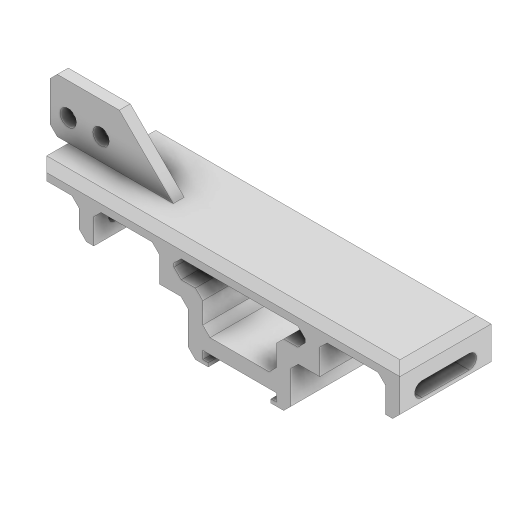
# Autodesk Inventor part: adapter_ver.1
Saved by Autodesk Inventor 2024 (Build 280153000, 153)
## iProperties
Created: 2023-11-09
Part Number: adapter_ver.1
Material: 一般
Document SubType Name: Modeling
Designer: moonshot
Density: 1 g/cm^3
Appearance: 既定
Author: moonshot
Autodesk Inventor part; units mm, degrees
ref_plane "YZ Plane" through (0, 0, 0) normal (1, 0, 0) x (0, 1, 0)
sketch "スケッチ1" plane through (0, 0, 0) normal (0, 0, 1) x (1, 0, 0)
  line L0 (94.5, 17.4061) -> (94.5, 4.4383)
  line L1 (64.6, 4.4061) -> (64.6, -8.5939)
  line L2 (36.4, -8.5939) -> (36.4, 4.4061)
  line L3 (0, -17.7867) -> (0, 46.5626) projected
  line L4 (40.4, -5.3939) -> (60.6, -5.3939)
  line L5 (64.6, -8.5939) -> (59.1, -8.5939)
  line L6 (41.9, -8.5939) -> (36.4, -8.5939)
  line L7 (72.5, 4.4061) -> (72.5, 13.4061)
  line L8 (72.5, 13.4061) -> (90.5, 13.4061)
  line L9 (90.5, 13.4061) -> (90.5, 4.4383)
  line L10 (50.5, -8.5617) -> (50.5, 17.1682) construction
  line L11 (28.5, 4.4061) -> (28.5, 13.4061)
  line L12 (28.5, 13.4061) -> (10.5, 13.4061)
  line L13 (10.5, 13.4061) -> (10.5, 4.4383)
  line L14 (0, 17.4061) -> (0, 13.4061)
  line L15 (0, 17.4061) -> (94.5, 17.4061)
  line L16 (94.5, 4.4383) -> (90.5, 4.4383)
  line L17 (72.5, 4.4061) -> (64.6, 4.4061)
  line L18 (6.5, 4.4383) -> (10.5, 4.4383)
  line L19 (28.5, 4.4061) -> (36.4, 4.4061)
  line L20 (6.5, 4.4383) -> (6.5, 13.4061)
  line L21 (6.5, 13.4061) -> (0, 13.4061)
  line L22 (72.5, 4.4061) -> (82.5, 4.4061) construction
  line L23 (82.5, 4.4061) -> (82.5, 13.4061) construction
  line L24 (77.5, 4.4061) -> (77.5, 37.3698) construction
  line L25 (28.5, 4.4061) -> (18.5, 4.4061) construction
  line L26 (18.5, 4.4061) -> (18.5, 13.4061) construction
  line L27 (23.5, 4.4061) -> (23.5, 33.4166) construction
  line L28 (41.9, -8.5939) -> (41.9, -7.5939)
  line L29 (41.9, -7.5939) -> (40.4, -7.5939)
  line L30 (40.4, -7.5939) -> (40.4, -5.3939)
  line L31 (59.1, -8.5939) -> (59.1, -7.5939)
  line L32 (59.1, -7.5939) -> (60.6, -7.5939)
  line L33 (60.6, -7.5939) -> (60.6, -5.3939)
  line L34 (32.5, 13.4061) -> (32.5, 8.4061)
  line L35 (40.4, 8.4061) -> (40.4, -1.3939)
  line L36 (40.4, -1.3939) -> (60.6, -1.3939)
  line L37 (60.6, -1.3939) -> (60.6, 8.4061)
  line L38 (60.6, 8.4061) -> (68.5, 8.4061)
  line L39 (68.5, 8.4061) -> (68.5, 13.4061)
  line L40 (68.5, 13.4061) -> (32.5, 13.4061)
  line L41 (32.5, 8.4061) -> (40.4, 8.4061)
  point P0 (0, 0)
  dimension "d10" = 20.2
  dimension "d14" = 18
  dimension "d18" = 13
  dimension "d23" = 4
  dimension "d40" = 4
  dimension "d41" = 9
  dimension "d42" = 10
  dimension "d43" = 10
  dimension "d44" = 50.5
  dimension "d74" = 4
  dimension "d78" = 1
  dimension "d79" = 2.2
  dimension "d80" = 1.5
  dimension "d81" = 1.5
  dimension "d82" = 1
  dimension "d83" = 23.5
  dimension "d84" = 4
  dimension "d86" = 4
  dimension "d87" = 4
  dimension "d88" = 4
  dimension "d89" = 4
  dimension "d90" = 4
  dimension "d91" = 4
  dimension "d92" = 4
  constraints: 82 end point, 23 perpendicular, 6 horizontal, 5 vertical, 4 symmetric about line, 3 point on line, 2 collinear, 2 midpoint, 2 other
  measures "d10" distance of L4.start L4.end
  measures "d14" distance of L7.end L8.end
  measures "d18" distance of L2.end L2.start
  measures "d23" distance between parallel lines of L0 L9
  measures "d40" distance of L18.start L13.end
  measures "d41" distance of L7.start L7.end
  measures "d42" distance of L7.start L22.end
  measures "d43" distance of L11.start L25.end
  measures "d44" distance between parallel lines of L10 L3
  measures "d74" distance between parallel lines of L21 L15
  measures "d78" distance of L6.start L28.end
  measures "d79" distance between parallel lines of L4 L29
  measures "d80" distance of L28.end L29.end
  measures "d81" distance of L31.end L32.end
  measures "d82" distance of L5.end L31.end
  measures "d83" distance between parallel lines of L27 L3
  measures "d84" distance between parallel lines of L30 L2
  measures "d86" distance between parallel lines of L11 L34
  measures "d87" distance between parallel lines of L2 L35
  measures "d88" distance between parallel lines of L4 L36
  measures "d89" distance between parallel lines of L1 L37
  measures "d90" distance between parallel lines of L7 L39
  measures "d91" distance between parallel lines of L17 L38
  measures "d92" distance between parallel lines of L19 L41
extrude "押し出し1" add sketch "スケッチ1" along normal mid plane 25
chamfer "面取り1" distance 2 angle 45 2 edges at (72.5, 13.4061, 0) (28.5, 13.4061, 0)
sketch "スケッチ4" plane through (94.5, 4.4383, 12.5) normal (1, 0, 0) x (0, 0, -1)
  line L0 (6, 3) -> (19, 3)
  arc A0 (19, 3) -> (19, 7) centre (19, 5) ccw
  line L1 (19, 7) -> (6, 7)
  arc A1 (6, 7) -> (6, 3) centre (6, 5) ccw
  line L2 (25, 12.9678) -> (25, 0) projected
  line L3 (0, 0) -> (0, 12.9678) projected
  line L4 (25, 0) -> (0, 0) projected
  point P0 (12.5, -4.4383)
  dimension "d45" = 4
  dimension "d46" = 6
  dimension "d47" = 6
  dimension "d48" = 3
  constraints: 4 end point, 4 point on circle, 4 tangent, 2 centre point, 2 horizontal
  measures "d45" distance between parallel lines of L0 L1
  measures "d46" distance from line of L2 A0.centre
  measures "d47" distance from line of L3 A1.centre
  measures "d48" distance between parallel lines of L4 L0
extrude "押し出し3" cut sketch "スケッチ4" against normal up to surface (4 mm away)
sketch "スケッチ5" plane through (6.5, 4.4383, 12.5) normal (-1, 0, 0) x (0, 0, 1)
  line L0 (-19, 3) -> (-6, 3) projected
  line L1 (-19, 3) -> (-6, 3)
  arc A0 (-6, 3) -> (-6, 7) centre (-6, 5) ccw
  line L2 (-6, 7) -> (-19, 7) projected
  line L3 (-6, 7) -> (-19, 7)
  arc A1 (-19, 7) -> (-19, 3) centre (-19, 5) ccw
  point P0 (-12.5, -4.4383)
  constraints: 4 end point, 4 point on circle, 4 tangent, 2 centre point, 2 equal length
extrude "押し出し4" cut sketch "スケッチ5" against normal up to surface (4 mm away)
chamfer "面取り4" distance 2 angle 45 20 edges at (90.5, 13.4061, 0) (10.5, 13.4061, 0) (6.5, 13.4061, 0) (64.6, 4.4061, 0) (36.4, 4.4061, 0) (40.4, 8.4061, 0) (32.5, 8.4061, 0) (32.5, 13.4061, 0) (68.5, 13.4061, 0) (68.5, 8.4061, 0) (60.6, 8.4061, 0) (60.6, -1.3939, 0) (40.4, -1.3939, 0) (36.4, -8.5939, 0) (64.6, -8.5939, 0) (94.5, 4.4383, 0) (94.5, 17.4061, 0) (47.25, 17.4061, 12.5) (47.25, 17.4061, -12.5) (6.5, 4.4383, 0)
ref_plane "作業平面1" through (0, 0, 1.5) normal (0, 0, 1) x (1, 0, 0)
sketch "スケッチ6" plane through (0, 0, 1.5) normal (0, 0, 1) x (1, 0, 0)
  line L0 (94.5, 17.4061) -> (0, 17.4061) projected
  line L1 (9.5, 17.4061) -> (-9.5, 17.4061)
  line L2 (-9.5, 17.4061) -> (-9.5, 32.2061)
  line L3 (-9.5, 32.2061) -> (9.5, 32.2061)
  line L4 (9.5, 32.2061) -> (9.5, 17.4061)
  line L5 (0, -5.8812) -> (0, 35.2873) projected
  circle A0 centre (4.5, 23.4061) radius 2.25
  circle A1 centre (-4.5, 23.4061) radius 2.25
  point P0 (0, 0)
  dimension "d57" = 19
  dimension "d58" = 14.8
  dimension "d59" = 4.5
  dimension "d60" = 4.5
  dimension "d61" = 6
  constraints: 8 end point, 3 perpendicular, 2 centre point, 1 collinear, 1 point on line, 1 symmetric about line, 2 other
  measures "d57" distance of L2.end L3.end
  measures "d58" distance of L1.end L2.end
  measures "d59" diameter of A0
  measures "d60" distance from line of L5 A0.centre
  measures "d61" distance from line of L0 A0.centre
extrude "押し出し5" add sketch "スケッチ6" along normal blind 3
ref_plane "作業平面2" through (0, 0, 0.1) normal (0, 0, 1) x (1, 0, 0)
sketch "スケッチ7" plane through (0, 0, 0.1) normal (0, 0, 1) x (1, 0, 0)
  line L0 (-9.5, 17.4061) -> (0, 17.4061) projected
  line L1 (9.5, 17.4061) -> (0, 17.4061) projected
  line L2 (9.5, 17.4061) -> (9.5, 32.2061) projected
  line L3 (9.5, 32.2061) -> (-9.5, 32.2061) projected
  line L4 (-9.5, 32.2061) -> (-9.5, 17.4061) projected
  circle A0 centre (4.5, 23.4061) radius 2.25 projected
  circle A1 centre (-4.5, 23.4061) radius 2.25 projected
  line L5 (0, 13.4061) -> (4.5, 13.4061) projected
  line L6 (0, 17.4061) -> (0, 13.4061) projected
  line L7 (0, 13.4061) -> (0, 17.4061)
  line L8 (0, 17.4061) -> (-9.5, 17.4061)
  line L9 (-9.5, 17.4061) -> (0, 17.4061) projected
  line L10 (-4.4, 13.4061) -> (0, 13.4061)
  line L11 (-4.4, 13.4061) -> (-4.4, 17.4061)
  point P0 (0, 0)
  dimension "d70" = 4.4
  constraints: 8 end point, 2 collinear, 1 perpendicular, 1 point on line
  measures "d70" distance of L10.start L5.start
extrude "押し出し6" add sketch "スケッチ7" along normal up to surface (12.4 mm away) contours L0 L6 L10 L11
chamfer "面取り5" distance 14.8 angle 45 1 edges at (9.5, 17.4061, 3)
sketch "スケッチ8" plane through (0, 0, -12.5) normal (0, 0, -1) x (-1, 0, 0)
  line L0 (-4.5, 13.4061) -> (4.4, 13.4061) projected
  line L1 (-0.05, 13.4061) -> (-4.5, 13.4061)
  line L2 (-4.5, 13.4061) -> (0, 13.4061) projected
  line L3 (0, 13.4061) -> (0, 15.4061) projected
  line L4 (-94.5, 15.4061) -> (-94.5, 6.4383) projected
  line L5 (-92.5, 4.4383) -> (-90.5, 4.4383) projected
  line L6 (-90.5, 4.4383) -> (-90.5, 11.4061) projected
  line L7 (-88.5, 13.4061) -> (-90.5, 11.4061) projected
  line L8 (-88.5, 13.4061) -> (-74.5, 13.4061) projected
  line L9 (-72.5, 11.4061) -> (-72.5, 4.4061) projected
  line L10 (-72.5, 4.4061) -> (-66.6, 4.4061) projected
  line L11 (-64.6, 2.4061) -> (-64.6, -6.5939) projected
  line L12 (-62.6, -8.5939) -> (-59.1, -8.5939) projected
  line L13 (-60.6, -5.3939) -> (-40.4, -5.3939) projected
  line L14 (-41.9, -8.5939) -> (-38.4, -8.5939) projected
  line L15 (-36.4, -6.5939) -> (-36.4, 2.4061) projected
  line L16 (-34.4, 4.4061) -> (-28.5, 4.4061) projected
  line L17 (-28.5, 4.4061) -> (-28.5, 11.4061) projected
  line L18 (-26.5, 13.4061) -> (-12.5, 13.4061) projected
  line L19 (-10.5, 11.4061) -> (-12.5, 13.4061) projected
  line L20 (-10.5, 11.4061) -> (-10.5, 4.4383) projected
  line L21 (-10.5, 4.4383) -> (-8.5, 4.4383) projected
  line L22 (-6.5, 6.4383) -> (-6.5, 11.4061) projected
  line L23 (-4.5, 13.4061) -> (-6.5, 11.4061) projected
  line L24 (-4.5, 13.4061) -> (-4.5, 17.4061)
  line L25 (0, 17.4061) -> (0, 13.4061)
  line L26 (0, 17.4061) -> (-4.5, 17.4061)
  line L27 (-59.1, -8.5939) -> (-59.1, -7.5939) projected
  line L28 (-59.1, -7.5939) -> (-60.6, -7.5939) projected
  line L29 (-60.6, -7.5939) -> (-60.6, -5.3939) projected
  line L30 (-40.4, -5.3939) -> (-40.4, -7.5939) projected
  line L31 (-40.4, -7.5939) -> (-41.9, -7.5939) projected
  line L32 (-41.9, -7.5939) -> (-41.9, -8.5939) projected
  line L33 (-72.5, 11.4061) -> (-74.5, 13.4061) projected
  line L34 (-26.5, 13.4061) -> (-28.5, 11.4061) projected
  line L35 (-64.6, 2.4061) -> (-66.6, 4.4061) projected
  line L36 (-34.4, 4.4061) -> (-36.4, 2.4061) projected
  line L37 (-62.6, -8.5939) -> (-64.6, -6.5939) projected
  line L38 (-36.4, -6.5939) -> (-38.4, -8.5939) projected
  line L39 (-6.5, 6.4383) -> (-8.5, 4.4383) projected
  line L40 (-94.5, 15.4061) -> (0, 15.4061) projected
  line L41 (-92.5, 4.4383) -> (-94.5, 6.4383) projected
  point P0 (0, 0)
  point P1 (4.5, 13.4383)
  point P2 (0, 13.4061)
  point P3 (-4.5, 15.4061)
  dimension "d71" = 4.45
  constraints: 8 end point, 1 horizontal, 1 perpendicular, 1 point on line, 1 vertical, 2 other
  measures "d71" distance of L1.start L1.end
extrude "押し出し7" cut sketch "スケッチ8" against normal blind 12.6 contours L24 L40 L3 L0 | L24 L26 L25 L40
chamfer "面取り7" distance 2 angle 45 6 edges at (-2.2, 17.4061, 12.5) (-4.4, 15.4061, 0.1) (-4.4, 15.4061, 12.5) (4.5, 14.4061, -12.5) (-9.5, 17.4061, 3) (-9.5, 32.2061, 3)
